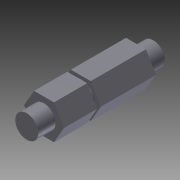
# Autodesk Inventor part: idler gear shaft
Saved by Autodesk Inventor 2012 (Build 160160000, 160)
## iProperties
Created: 2012-02-21
Part Number: idler gear shaft
Material: Steel
Document SubType Name: Modeling
Designer: Antonella Wilby
Mass: 15.6662 g
Surface Area: 9.95229 cm^2
Volume: 1.9957 cm^3
Density: 7.85 g/cm^3
Author: Antonella Wilby
Autodesk Inventor part; units mm, degrees
ref_plane "YZ Plane" through (0, 0, 0) normal (1, 0, 0) x (0, 1, 0)
ref_plane "XZ Plane" through (0, 0, 0) normal (0, 1, 0) x (-1, 0, 0)
sketch "Sketch1" plane through (0, 0, 0) normal (0, 0, 1) x (1, 0, 0)
  line L0 (2.7496, 4.7625) -> (5.4993, 0)
  line L1 (5.4993, 0) -> (2.7496, -4.7625)
  line L2 (2.7496, -4.7625) -> (-2.7496, -4.7625)
  line L3 (-2.7496, -4.7625) -> (-5.4993, 0)
  line L4 (-5.4993, 0) -> (-2.7496, 4.7625)
  line L5 (-2.7496, 4.7625) -> (2.7496, 4.7625)
  point P0 (0, 0)
  point P1 (0, 0)
  point P2 (0, 4.7625)
  dimension "d0" = 9.525
  constraints: 12 end point, 1 coincident, 1 midpoint, 1 vertical alignment, 13 other
  measures "d0" distance between parallel lines of L5 L2
extrude "Extrusion1" add sketch "Sketch1" along normal mid plane 34.925
sketch "Sketch2" plane through (0, 0, 17.4625) normal (0, 0, 1) x (1, 0, 0)
  line L0 (5.4993, 0) -> (2.7496, -4.7625) projected
  line L1 (2.7496, 4.7625) -> (5.4993, 0) projected
  line L2 (-2.7496, 4.7625) -> (2.7496, 4.7625) projected
  line L3 (-5.4993, 0) -> (-2.7496, 4.7625) projected
  line L4 (-2.7496, -4.7625) -> (-5.4993, 0) projected
  line L5 (2.7496, -4.7625) -> (-2.7496, -4.7625) projected
  circle A0 centre (0, 0) radius 3.175
  dimension "d3" = 6.35
  constraints: 1 centre point, 1 coincident
  measures "d3" diameter of A0
extrude "Extrusion2" cut sketch "Sketch2" against normal blind 4.7625
mirror "Mirror1" about plane through (0, 0, 0) normal (0, 0, 1) of "Extrusion2"
ref_plane "Work Plane1" through (0, 0, 2.54) normal (0, 0, 1) x (1, 0, 0)
sketch "Sketch3" plane through (0, 0, 2.54) normal (0, 0, 1) x (1, 0, 0)
  circle A0 centre (0, 0) radius 3.175 projected
  line L0 (2.7496, 4.7625) -> (5.4993, 0) projected
  line L1 (-2.7496, 4.7625) -> (2.7496, 4.7625) projected
  line L2 (-5.4993, 0) -> (-2.7496, 4.7625) projected
  line L3 (-2.7496, -4.7625) -> (-5.4993, 0) projected
  line L4 (2.7496, -4.7625) -> (-2.7496, -4.7625) projected
  line L5 (5.4993, 0) -> (2.7496, -4.7625) projected
  line L6 (-2.7496, 4.7625) -> (2.7496, 4.7625) projected
  line L7 (-5.4993, 0) -> (-2.7496, 4.7625) projected
  line L8 (-2.7496, -4.7625) -> (-5.4993, 0) projected
  line L9 (2.7496, -4.7625) -> (-2.7496, -4.7625) projected
  line L10 (5.4993, 0) -> (2.7496, -4.7625) projected
  line L11 (2.7496, 4.7625) -> (5.4993, 0) projected
  circle A1 centre (0, 0) radius 3.8481
  point P0 (0, 0)
  dimension "d8" = 7.6962
  constraints: 1 centre point, 1 coincident
  measures "d8" diameter of A1
extrude "E-clip Groove" cut sketch "Sketch3" along normal blind 0.9906 contours L0 L5 L4 L3 L2 L1
body "Solid1"
